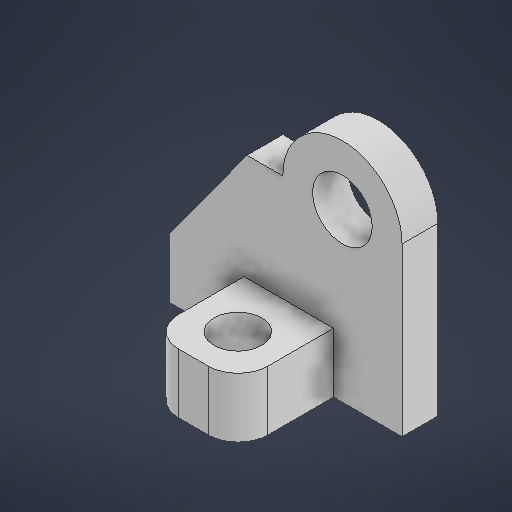
# Autodesk Inventor part: Prova1
Saved by Autodesk Inventor 2026.3 (Build 303398000, 398)
## iProperties
Created: 2026-05-17
Part Number: Prova1
Material: Genérico
Document SubType Name: Modeling
Designer: alenc
Density: 1 g/cm^3
Appearance: Padrão
Author: alenc
Autodesk Inventor part; units mm, degrees
ref_plane "YZ Plane" through (0, 0, 0) normal (1, 0, 0) x (0, 1, 0)
ref_plane "XZ Plane" through (0, 0, 0) normal (0, 1, 0) x (-1, 0, 0)
ref_plane "XY Plane" through (0, 0, 0) normal (0, 0, 1) x (1, 0, 0)
sketch "Esboço1" plane through (0, 0, 0) normal (0, 0, 1) x (1, 0, 0)
  line L0 (19.5, -14) -> (19.5, 14)
  line L1 (-19.5, -14) -> (19.5, 14) construction
  line L2 (19.5, -14) -> (-19.5, 14) construction
  circle A0 centre (9.5, 14) radius 10
  circle A1 centre (9.5, 14) radius 5
  line L3 (-19.5, -14) -> (-19.5, -4)
  line L4 (-0.4993, 13.8849) -> (-6.4993, 13.8849)
  line L5 (-19.5, -4) -> (-6.4993, 13.8849)
  line L6 (-19.5, -14) -> (-7, -14)
  line L7 (-7, -14) -> (-7, -4)
  line L8 (-7, -4) -> (8, -4)
  line L9 (8, -4) -> (8, -14)
  line L10 (8, -14) -> (19.5, -14)
  line L11 (-7, -14) -> (8, -14)
  point P0 (0, 0)
  dimension "d0" = 28
  dimension "d2" = 20
  dimension "d3" = 10
  dimension "d5" = 10
  dimension "d6" = 6
  dimension "d8" = 12.5
  dimension "d9" = 15
  dimension "d10" = 10
  dimension "d11" = 10
  dimension "d12" = 15
  dimension "d13" = 11.5
  dimension "d14" = 22.1107
  constraints: 24 end point, 3 horizontal, 3 perpendicular, 2 centre point, 2 midpoint, 2 point on circle, 2 point on line, 1 coincident, 1 vertical
  measures "d0" distance of L0.start L0.end
  measures "d2" diameter of A0
  measures "d3" diameter of A1
  measures "d5" distance of L1.start L3.end
  measures "d6" distance of L4.start L4.end
  measures "d8" distance of L1.start L6.end
  measures "d9" distance of L6.end L9.end
  measures "d10" distance of L6.end L7.end
  measures "d11" distance of L8.end L9.end
  measures "d12" distance of L7.end L8.end
  measures "d13" distance of L9.end L10.end
  measures "d14" distance of L3.end L4.end
extrude "Extrusão1" add sketch "Esboço1" along normal blind 6
sketch "Esboço2" plane through (0, 0, 6) normal (0, 0, 1) x (1, 0, 0)
  line L0 (-7, -14) -> (-7, -4)
  line L1 (-7, -4) -> (8, -4)
  line L2 (8, -4) -> (8, -14)
  line L3 (-19.5, -4) -> (-19.5, -14) projected
  line L4 (-19.5, -14) -> (-7, -14)
  line L5 (-7, -14) -> (8, -14)
  line L6 (8, -14) -> (18.5, -14)
  point P0 (0, 0)
  dimension "d17" = 90
  dimension "d18" = 10
  dimension "d19" = 15
  dimension "d20" = 12.5
  dimension "d21" = 10.5
  dimension "d22" = 15
  constraints: 12 end point, 3 perpendicular, 1 collinear, 1 point on line, 1 vertical
  measures "d17" angle of L2 L6
  measures "d18" distance of L1.end L2.end
  measures "d19" distance of L0.end L1.end
  measures "d20" distance of L0.start L3.end
  measures "d21" distance from line of L6.end L2
  measures "d22" distance of L2.end L0.start
extrude "Extrusão2" add sketch "Esboço2" along normal blind 16
sketch "Esboço3" plane through (-7, -4, 6) normal (0, 1, 0) x (1, 0, 0)
  circle A0 centre (7.4721, -8.5158) radius 4
  point P0 (7, 6)
  dimension "d25" = 8
  constraints: 1 centre point
  measures "d25" diameter of A0
fillet "Arredondamento1" radius 5 2 edges at (8, -9, 22) (-7, -9, 22)
hole "Furo1" at (0.4721, -4, 14.5158) direction (0, -1, 0) diameter 8 end through all
